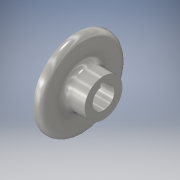
# Autodesk Inventor part: Brida de la Rueda
Saved by Autodesk Inventor 2016 (Build 200138000, 138)
## iProperties
Created: 2016-05-05
Part Number: Brida de la Rueda
Material: Aluminum 6061-AHC
Document SubType Name: Modeling
Designer: Jorge
Density: 2.7 g/cm^3
Appearance: Aluminum - Dark
Mass: 25.02 g
Surface Area: 57.0788 cm^2
Volume: 9.26667 cm^3
Author: Jorge
Title: Brida de la Rueda
Autodesk Inventor part; units mm, degrees
ref_plane "YZ Plane" through (0, 0, 0) normal (1, 0, 0) x (0, 1, 0)
ref_plane "XZ Plane" through (0, 0, 0) normal (0, 1, 0) x (-1, 0, 0)
ref_plane "XY Plane" through (0, 0, 0) normal (0, 0, 1) x (1, 0, 0)
sketch "Sketch1" plane through (0, 0, 0) normal (0, 0, 1) x (1, 0, 0)
  line L0 (0, 25.4) -> (0.7937, 25.4)
  line L1 (3.9687, 22.225) -> (3.9688, 14.2875)
  line L2 (7.1437, 11.1125) -> (15.875, 11.1125)
  line L3 (0, 25.4) -> (0, 22.225)
  line L4 (-3.175, 0) -> (19.05, 0) projected
  line L5 (0, -5.2115) -> (0, 31.2691) construction
  line L6 (15.875, 11.1125) -> (15.875, 6.35)
  arc A0 (3.9687, 22.225) -> (0.7937, 25.4) centre (0.7937, 22.225) ccw
  arc A1 (3.9688, 14.2875) -> (7.1437, 11.1125) centre (7.1438, 14.2875) ccw
  line L7 (0.7937, 22.225) -> (0.7937, 6.35)
  line L8 (0.7937, 22.225) -> (0, 22.225)
  line L9 (0.7937, 6.35) -> (15.875, 6.35)
  point P0 (0, 0)
  dimension "d0" = 50.8
  dimension "d1" = 22.225
  dimension "d2" = 0
  dimension "d3" = 15.875
  dimension "d4" = 3.9688
  dimension "d5" = 3.175
  dimension "d6" = 0.7937
  dimension "d7" = 44.45
  dimension "d8" = 12.7
  constraints: 16 end point, 4 point on circle, 4 tangent, 3 perpendicular, 3 vertical, 2 centre point, 2 horizontal, 1 equal radius
  measures "d0" diameter of L0 L4
  measures "d1" diameter of L2 L4
  measures "d2" distance between parallel lines of L5 L3
  measures "d3" distance between parallel lines of L6 L3
  measures "d4" distance between parallel lines of L3 L1
  measures "d5" radius of A0
  measures "d6" distance between parallel lines of L3 L7
  measures "d7" diameter of L8 L4
  measures "d8" diameter of L9 L4
revolve "Revolution1" add sketch "Sketch1" angle 360 about axis through (-10, 0, 0) along (1, 0, 0)
sketch "Sketch2" plane through (15.875, 0, 0) normal (1, 0, 0) x (0, 0, -1)
  line L0 (0, -35.56) -> (0, 35.56) construction
  line L1 (35.56, 0) -> (-35.56, 0) construction
  line L2 (-1.5875, 7.9375) -> (1.5875, 7.9375)
  line L3 (1.5875, 7.9375) -> (1.5875, 4.7625)
  line L4 (1.5875, 4.7625) -> (-1.5875, 4.7625)
  line L5 (-1.5875, 4.7625) -> (-1.5875, 7.9375)
  line L6 (-4.6004, 6.35) -> (6.3294, 6.35) construction
  circle A0 centre (0, 0) radius 6.35 construction
  dimension "d10" = 3.175
  dimension "d11" = 1.5875
  dimension "d12" = 1.5875
  dimension "d13" = 3.175
  constraints: 10 end point, 2 horizontal, 2 parallel, 1 perpendicular, 1 tangent
  measures "d10" distance between parallel lines of L5 L3
  measures "d11" distance between parallel lines of L0 L5
  measures "d12" distance between parallel lines of L2 L6
  measures "d13" distance between parallel lines of L2 L4
extrude "Extrusion1" cut sketch "Sketch2" against normal through all
equation "\"d11\" = 0.5 * d10"
equation "\"d13\" = 2 * d12"
body "Solid1"
